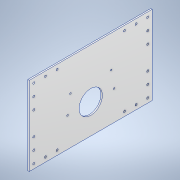
# Autodesk Inventor part: ODSY-0007-001
Saved by Autodesk Inventor 2021 (Build 250183000, 183)
## iProperties
Company: ERPL
Created: 2021-09-11
Material: Aluminum 6061
Document SubType Name: Modeling
Designer: ALEX CLAY
Density: 2.7 g/cm^3
Appearance: Aluminum - Flat
Mass: 3003.69 g
Surface Area: 3691.99 cm^2
Volume: 1112.48 cm^3
Project: ODYSSEY
Description: ODYSSEY THRUST PLATE
Part Number: ODSY-0007-001
Author: ALEX CLAY
Revision Number: 00
Autodesk Inventor part; units mm, degrees
ref_plane "YZ Plane" through (0, 0, 0) normal (1, 0, 0) x (0, 1, 0)
ref_plane "XZ Plane" through (0, 0, 0) normal (0, 1, 0) x (-1, 0, 0)
ref_plane "XY Plane" through (0, 0, 0) normal (0, 0, 1) x (1, 0, 0)
sketch "Sketch1" plane through (0, 0, 0) normal (1, 0, 0) x (0, 1, 0)
  line L0 (-172.4, 268.6) -> (172.4, 268.6)
  line L1 (172.4, 268.6) -> (172.4, -268.6)
  line L2 (172.4, -268.6) -> (-172.4, -268.6)
  line L3 (-172.4, -268.6) -> (-172.4, 268.6)
  point P0 (0, 0)
  dimension "d0" = 537.2
  dimension "d1" = 344.8
  dimension "d96" = 268.6
  dimension "d97" = 172.4
  constraints: 8 end point, 2 parallel, 1 horizontal, 1 perpendicular
  measures "d0" distance of L0.end L1.end
  measures "d1" distance of L1.end L2.end
  measures "d96" distance from line of L2 point (0, 0)
  measures "d97" distance from line of point (0, 0) L1
extrude "Extrusion1" add sketch "Sketch1" along normal blind 6.35
sketch "Sketch2" plane through (6.35, 0, 0) normal (1, 0, 0) x (0, 0, -1)
  circle A0 centre (-0.005, -43.5) radius 50.8
  line L0 (-268.6, 172.4) -> (-268.6, -172.4) projected
  line L1 (268.6, -172.4) -> (268.6, 172.4) projected
  line L2 (268.6, 172.4) -> (-268.6, 172.4) projected
  line L3 (-268.6, -172.4) -> (268.6, -172.4) projected
  dimension "d6" = 101.6
  dimension "d51" = 268.605
  dimension "d65" = 215.9
  constraints: 1 centre point
  measures "d6" diameter of A0
  measures "d51" distance from line of L1 A0.centre
  measures "d65" distance from line of L2 A0.centre
extrude "Extrusion2" cut sketch "Sketch2" against normal through all contours A0
sketch "Sketch5" plane through (6.35, 0, 0) normal (1, 0, 0) x (0, 0, -1)
  line L0 (-101.6, -43.5) -> (101.6, -43.5) construction
  circle A0 centre (-0.005, -43.5) radius 37.8815 construction
  circle A1 centre (-0.005, -43.5) radius 50.8 projected
  point P0 (0, 0)
  dimension "d62" = 203.2
  dimension "d63" = 101.6
  dimension "d64" = 75.7631
  constraints: 2 end point, 1 centre point, 1 concentric, 1 horizontal, 1 point on line
  measures "d62" distance of L0.start L0.end
  measures "d63" horizontal distance of L0.start point (0, 0)
  measures "d64" diameter of A0
hole "Hole1" at (6.35, -43.5, 101.6) at (6.35, -43.5, -101.6) direction (-1, 0, 0) diameter 7.1374 end through all clearance for "Socket Head Cap Screw" size "1/4" standard "Ansi Unified Screw Threads"
sketch "Sketch6" plane through (6.35, 0, 0) normal (1, 0, 0) x (0, 0, -1)
  line L0 (-88.9, 32.7) -> (88.9, 32.7) construction
  circle A0 centre (-0.005, -43.5) radius 50.8 projected
  point P0 (0, 0)
  dimension "d73" = 177.8
  dimension "d75" = 88.9
  dimension "d76" = 76.2
  constraints: 2 end point, 1 horizontal
  measures "d73" distance of L0.start L0.end
  measures "d75" horizontal distance of point (0, 0) L0.start
  measures "d76" vertical distance of A0.centre L0.start
hole "Hole2" at (6.35, 32.7, 88.9) at (6.35, 32.7, -88.9) direction (-1, 0, 0) diameter 6.7564 end through all clearance for "Socket Head Cap Screw" size "1/4" standard "Ansi Unified Screw Threads"
sketch "Sketch7" plane through (6.35, 0, 0) normal (1, 0, 0) x (0, 0, -1)
  line L0 (268.6, 172.4) -> (-268.6, 172.4) projected
  line L1 (-268.6, 172.4) -> (-268.6, -172.4) projected
  line L2 (-268.6, -172.4) -> (268.6, -172.4) projected
  point P0 (0, 0)
  point P1 (-248.6, 152.4)
  point P2 (-248.6, 101.6)
  point P3 (-197.8, 152.4)
  point P4 (-147, 152.4)
  point P5 (-248.6, 50.8)
  point P6 (-248.6, -50.8)
  point P7 (-248.6, -101.6)
  point P8 (-248.6, -152.4)
  point P9 (-197.8, -152.4)
  point P10 (-147, -152.4)
  dimension "d84" = 20
  dimension "d85" = 20
  dimension "d86" = 50.8
  dimension "d87" = 50.8
  dimension "d88" = 50.8
  dimension "d89" = 50.8
  dimension "d90" = 20
  dimension "d91" = 20
  dimension "d92" = 50.8
  dimension "d93" = 50.8
  dimension "d94" = 50.8
  dimension "d95" = 50.8
  constraints: 4 horizontal alignment, 4 vertical alignment
  measures "d84" distance from line of point (-248.6, 152.4) L0
  measures "d85" distance from line of point (-248.6, 152.4) L1
  measures "d86" distance of point (-248.6, 101.6) point (-248.6, 152.4)
  measures "d87" distance of point (-248.6, 101.6) point (-248.6, 50.8)
  measures "d88" distance of point (-248.6, 152.4) point (-197.8, 152.4)
  measures "d89" distance of point (-147, 152.4) point (-197.8, 152.4)
  measures "d90" distance from line of L2 point (-248.6, -152.4)
  measures "d91" distance from line of L1 point (-248.6, -152.4)
  measures "d92" distance of point (-248.6, -152.4) point (-197.8, -152.4)
  measures "d93" distance of point (-197.8, -152.4) point (-147, -152.4)
  measures "d94" distance of point (-248.6, -101.6) point (-248.6, -152.4)
  measures "d95" distance of point (-248.6, -101.6) point (-248.6, -50.8)
hole "Hole3" at (6.35, 152.4, 248.6) at (6.35, 101.6, 248.6) at (6.35, 152.4, 197.8) at (6.35, 152.4, 147) at (6.35, 50.8, 248.6) at (6.35, -50.8, 248.6) at (6.35, -101.6, 248.6) at (6.35, -152.4, 248.6) at (6.35, -152.4, 197.8) at (6.35, -152.4, 147) direction (-1, 0, 0) diameter 8.9916 end through all clearance for "Socket Head Cap Screw" size "M8" standard "Ansi Metric M Profile"
mirror "Mirror1" about plane through (0, 0, 0) normal (0, 0, 1) of "Hole3"
equation "\"d96\" = 0.5 * d0"
equation "\"d97\" = 0.5 * d1"
equation "\"d75\" = 0.5 * d73"
equation "\"d93\" = d92"
equation "\"d94\" = d92"
equation "\"d95\" = d94"
body "Solid1"
